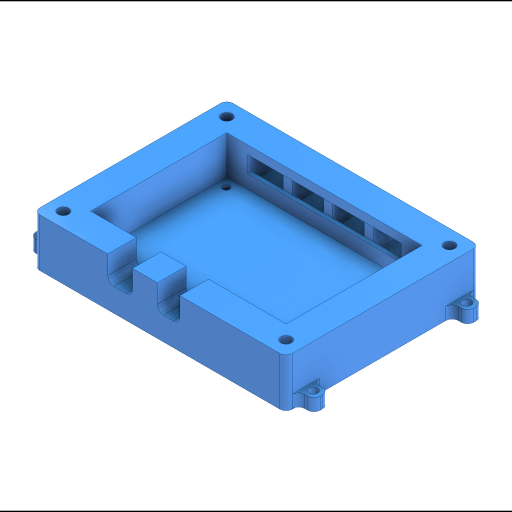
# Autodesk Inventor part: PowerBoardCase
Saved by Autodesk Inventor 2023 (Build 270158000, 158)
## iProperties
Created: 2022-02-06
Part Number: PowerBoardCase
Material: Generic
Document SubType Name: Modeling
Designer: kamer
Density: 1 g/cm^3
Appearance: Cyan
Author: kamer
## iProperties of the stored document _3DPrint.ipt
Created: 2022-02-06
Part Number: _3DPrint
Material: Generic
Document SubType Name: Modeling
Designer: kamer
Density: 1 g/cm^3
Appearance: Default
Author: kamer
Autodesk Inventor part; units mm, degrees
ref_plane "YZ Plane" through (0, 0, 0) normal (1, 0, 0) x (0, 1, 0)
ref_plane "XZ Plane" through (0, 0, 0) normal (0, 1, 0) x (-1, 0, 0)
ref_plane "XY Plane" through (0, 0, 0) normal (0, 0, 1) x (1, 0, 0)
sketch "Sketch1" plane through (0, 0, 0) normal (0, 1, 0) x (-1, 0, 0)
  line L0 (0, 0) -> (-100.33, 0)
  line L1 (-100.33, 0) -> (-100.33, -69.85)
  line L2 (-100.33, -69.85) -> (0, -69.85)
  line L3 (0, -69.85) -> (0, 0)
  line L4 (2, -71.85) -> (-102.33, -71.85)
  line L5 (-102.33, -71.85) -> (-102.33, 2)
  line L6 (-102.33, 2) -> (2, 2)
  line L7 (2, 2) -> (2, -71.85)
  dimension "d0" = 100.33
  dimension "d1" = 69.85
  dimension "d3" = 2
  dimension "d4" = 2
  dimension "d5" = 2
  dimension "d6" = 2
  constraints: 16 end point, 4 parallel, 2 horizontal, 2 perpendicular
  measures "d0" distance of L2.end L1.end
  measures "d1" distance of L1.end L0.end
  measures "d3" distance between parallel lines of L2 L4
  measures "d4" distance between parallel lines of L1 L5
  measures "d5" distance between parallel lines of L7 L3
  measures "d6" distance between parallel lines of L0 L6
extrude "Extrusion1" add sketch "Sketch1" along normal blind 7.112
sketch "Sketch2" plane through (0, 0, 0) normal (0, -1, 0) x (1, 0, 0)
  line L0 (-2, 2) -> (102.33, 2) projected
  line L1 (-2, -71.85) -> (-2, 2) projected
  line L2 (102.33, -71.85) -> (-2, -71.85) projected
  line L3 (102.33, 2) -> (102.33, -71.85) projected
  line L4 (100.33, 0) -> (0, 0) projected
  line L5 (100.33, -69.85) -> (100.33, 0) projected
  line L6 (0, -69.85) -> (100.33, -69.85) projected
  line L7 (0, 0) -> (0, -69.85) projected
extrude "Extrusion2" add sketch "Sketch2" along normal blind 5 contours L0 L3 L2 L1 | L5 L6 L7 L4
sketch "Sketch3" plane through (0, -5, 0) normal (0, -1, 0) x (1, 0, 0)
  circle A0 centre (96.4565, -65.183) radius 3.81
  circle A1 centre (4.3815, -65.183) radius 3.81
  circle A2 centre (4.3754, -4.858) radius 3.81
  circle A3 centre (96.4504, -4.858) radius 3.81
  line L0 (-2, 2) -> (-2, -71.85) projected
  line L1 (102.33, 2) -> (-2, 2) projected
  point P0 (0, 0)
  dimension "d11" = 7.62
  dimension "d12" = 7.62
  dimension "d13" = 7.62
  dimension "d14" = 7.62
  dimension "d15" = 60.325
  dimension "d16" = 60.325
  dimension "d17" = 0
  dimension "d18" = 92.075
  dimension "d19" = 92.075
  dimension "d20" = 6.3815
  dimension "d21" = 6.3754
  dimension "d22" = 6.858
  constraints: 4 centre point
  measures "d11" diameter of A0
  measures "d12" diameter of A1
  measures "d13" diameter of A2
  measures "d14" diameter of A3
  measures "d15" distance of A3.centre A0.centre
  measures "d16" distance of A2.centre A1.centre
  measures "d17" vertical distance of A1.centre A0.centre
  measures "d18" distance of A1.centre A0.centre
  measures "d19" distance of A2.centre A3.centre
  measures "d20" distance from line of A1.centre L0
  measures "d21" distance from line of L0 A2.centre
  measures "d22" distance from line of L1 A2.centre
extrude "Extrusion3" cut sketch "Sketch3" against normal blind 3.8
sketch "Sketch4" plane through (96.4565, -1.2, -65.183) normal (0, -1, 0) x (1, 0, 0)
  circle A0 centre (0, 0) radius 3.81 projected
  circle A1 centre (-0.0061, 60.325) radius 3.81 projected
  circle A2 centre (-92.0811, 60.325) radius 3.81 projected
  circle A3 centre (-92.075, 0) radius 3.81 projected
  circle A4 centre (0, 0) radius 1.778
  circle A5 centre (-92.075, 0) radius 1.778
  circle A6 centre (-92.0811, 60.325) radius 1.778
  circle A7 centre (-0.0061, 60.325) radius 1.778
  point P0 (-96.4565, 65.183)
  dimension "d25" = 3.556
  dimension "d26" = 3.556
  dimension "d27" = 3.556
  dimension "d28" = 3.556
  constraints: 4 centre point, 4 coincident
  measures "d25" diameter of A4
  measures "d26" diameter of A5
  measures "d27" diameter of A6
  measures "d28" diameter of A7
extrude "Extrusion4" cut sketch "Sketch4" against normal through all contours A4 | A5 | A6 | A7
sketch "Sketch5" plane through (0, 0, 0) normal (0, 1, 0) x (1, 0, 0)
  line L0 (9.525, 60.325) -> (90.805, 60.325)
  line L1 (90.805, 60.325) -> (90.805, 9.525)
  line L2 (90.805, 9.525) -> (9.525, 9.525)
  line L3 (9.525, 9.525) -> (9.525, 60.325)
  line L4 (0, 0) -> (0, 69.85) projected
  line L5 (0, 69.85) -> (100.33, 69.85) projected
  line L6 (100.33, 69.85) -> (100.33, 0) projected
  line L7 (100.33, 0) -> (0, 0) projected
  dimension "d31" = 9.525
  dimension "d32" = 9.525
  dimension "d33" = 9.525
  dimension "d34" = 9.525
  constraints: 8 end point, 2 parallel, 1 horizontal, 1 perpendicular
  measures "d31" distance between parallel lines of L4 L3
  measures "d32" distance between parallel lines of L5 L0
  measures "d33" distance between parallel lines of L6 L1
  measures "d34" distance between parallel lines of L7 L2
extrude "Extrusion5" cut sketch "Sketch5" against normal through all contours L0 L1 L2 L3
sketch "Sketch6" plane through (0, 7.112, 0) normal (0, 1, 0) x (1, 0, 0)
  line L0 (-2, -2) -> (102.33, -2) projected
  line L1 (102.33, -2) -> (102.33, 71.85) projected
  line L2 (102.33, 71.85) -> (-2, 71.85) projected
  line L3 (-2, 71.85) -> (-2, -2) projected
  line L4 (100.33, 0) -> (0, 0) projected
  line L5 (0, 0) -> (0, 69.85) projected
  line L6 (0, 69.85) -> (100.33, 69.85) projected
  line L7 (100.33, 69.85) -> (100.33, 0) projected
  line L8 (-2, 71.85) -> (102.33, 71.85) projected
  line L9 (0, 69.85) -> (100.33, 69.85) projected
  line L10 (10.7, 71.85) -> (89.63, 71.85)
  line L11 (89.63, 71.85) -> (89.63, 69.85)
  line L12 (89.63, 69.85) -> (10.7, 69.85)
  line L13 (10.7, 69.85) -> (10.7, 71.85)
  line L14 (100.33, 0) -> (0, 0) projected
  line L15 (23.4, 0) -> (36.1, 0)
  line L16 (36.1, 0) -> (36.1, -2)
  line L17 (36.1, -2) -> (23.4, -2)
  line L18 (23.4, -2) -> (23.4, 0)
  line L19 (48.99, 0) -> (60.42, 0)
  line L20 (60.42, 0) -> (60.42, -2)
  line L21 (60.42, -2) -> (48.99, -2)
  line L22 (48.99, -2) -> (48.99, 0)
  point P0 (10.7, 69.85)
  dimension "d37" = 12.7
  dimension "d38" = 12.7
  dimension "d39" = 12.7
  dimension "d40" = 25.4
  dimension "d41" = 41.91
  dimension "d42" = 11.43
  constraints: 24 end point, 6 parallel, 6 point on line, 3 horizontal, 3 perpendicular
  measures "d37" distance between parallel lines of L3 L13
  measures "d38" distance between parallel lines of L1 L11
  measures "d39" distance between parallel lines of L16 L18
  measures "d40" distance between parallel lines of L3 L18
  measures "d41" distance between parallel lines of L1 L20
  measures "d42" distance between parallel lines of L22 L20
extrude "Extrusion6" add sketch "Sketch6" along normal blind 12.7 contours L3 L2 L13 L6 L5 L4 L18 L0 | L16 L4 L22 L0 | L2 L1 L0 L20 L4 L7 L6 L11
sketch "Sketch7" plane through (9.525, 0, -9.525) normal (1, 0, 0) x (0, 0, -1)
  line L0 (50.8, -5) -> (0, -5) projected
  line L1 (50.8, 0) -> (50.8, -5) projected
  line L2 (0, 0) -> (50.8, 0) projected
  line L3 (0, 0) -> (0, -5) projected
  point P0 (-9.525, 0)
extrude "Extrusion7" add sketch "Sketch7" along normal up to surface (81.28 mm away)
sketch "Sketch12" plane through (102.33, -5, 2) normal (1, 0, 0) x (0, 0, -1)
  line L0 (0, 0) -> (0, 24.812) projected
  line L1 (73.85, 0) -> (73.85, 24.812) projected
  line L2 (0, 24.812) -> (73.85, 24.812)
  line L3 (73.85, 24.812) -> (73.85, 0)
  line L4 (73.85, 0) -> (0, 0)
  line L5 (0, 0) -> (0, 24.812)
  point P0 (2, 5)
  constraints: 8 end point, 2 parallel, 1 horizontal, 1 perpendicular
extrude "Extrusion12" add sketch "Sketch12" along normal blind 12.7
sketch "Sketch13" plane through (-2, -5, -71.85) normal (-1, 0, 0) x (0, 0, 1)
  line L0 (73.85, 24.812) -> (73.85, 0) projected
  line L1 (0, 24.812) -> (73.85, 24.812) projected
  line L2 (0, 0) -> (0, 24.812) projected
  line L3 (73.85, 0) -> (0, 0) projected
  point P0 (71.85, 5)
extrude "Extrusion13" add sketch "Sketch13" along normal blind 12.7
sketch "Sketch14" plane through (36.1, 19.812, 2) normal (0, 0, 1) x (1, 0, 0)
  line L0 (24.32, 0) -> (78.93, 0) projected
  line L1 (24.32, -12.7) -> (24.32, 0) projected
  line L2 (12.89, -12.7) -> (24.32, -12.7) projected
  line L3 (12.89, -12.7) -> (12.89, 0) projected
  line L4 (0, 0) -> (12.89, 0) projected
  line L5 (0, -12.7) -> (0, 0) projected
  line L6 (-12.7, -12.7) -> (0, -12.7) projected
  line L7 (-12.7, -12.7) -> (-12.7, 0) projected
  line L8 (-12.7, 0) -> (-50.8, 0) projected
  line L9 (-50.8, -24.812) -> (-50.8, 0) projected
  line L10 (-50.8, -24.812) -> (78.93, -24.812) projected
  line L11 (78.93, 0) -> (78.93, -24.812) projected
  point P0 (-36.1, -19.812)
extrude "Extrusion14" add sketch "Sketch14" along normal blind 12.7
sketch "Sketch16" plane through (89.63, 7.112, -71.85) normal (0, 0, -1) x (-1, 0, 0)
  line L0 (78.93, 12.7) -> (104.33, 12.7) projected
  line L1 (78.93, 0) -> (78.93, 12.7) projected
  line L2 (0, 0) -> (78.93, 0) projected
  line L3 (0, 0) -> (0, 12.7) projected
  line L4 (0, 12.7) -> (-25.4, 12.7) projected
  line L5 (-25.4, -12.112) -> (-25.4, 12.7) projected
  line L6 (-25.4, -12.112) -> (104.33, -12.112) projected
  line L7 (104.33, 12.7) -> (104.33, -12.112) projected
  line L8 (78.93, 0) -> (0, 0) projected
  line L9 (0, 0) -> (78.93, 0)
  line L10 (78.93, 0) -> (78.93, -4.492)
  line L11 (78.93, -4.492) -> (0, -4.492)
  line L12 (0, -4.492) -> (0, 0)
  point P0 (89.63, -7.112)
  dimension "d86" = 7.62
  constraints: 8 end point, 2 parallel, 1 horizontal, 1 perpendicular
  measures "d86" distance between parallel lines of L6 L11
extrude "Extrusion16" add sketch "Sketch16" along normal blind 12.7 contours L0 L7 L6 L5 L4 L3 L12 L11 L10 L1
sketch "Sketch17" plane through (0, 19.812, 0) normal (0, 1, 0) x (1, 0, 0)
  point P0 (0, 0)
sketch "Sketch18" plane through (89.63, 7.112, -71.85) normal (-1, 0, 0) x (0, 0, 1)
  line L0 (-12.7, -4.492) -> (-12.7, 12.7) projected
  line L1 (2, 0) -> (2, 12.7) projected
  line L2 (-12.7, 12.7) -> (2, 12.7)
  line L3 (2, 12.7) -> (2, 8.382)
  line L4 (2, 8.382) -> (-12.7, 8.382)
  line L5 (-12.7, 8.382) -> (-12.7, 12.7)
  point P0 (71.85, -7.112)
  point P1 (-12.7, 8.382)
  dimension "d89" = 4.318
  constraints: 8 end point, 2 parallel, 1 horizontal, 1 perpendicular, 1 point on line
  measures "d89" distance between parallel lines of L2 L4
extrude "Extrusion17" add sketch "Sketch18" along normal up to surface (78.93 mm away)
sketch "Sketch19" plane through (89.63, 7.112, -71.85) normal (0, 0, -1) x (-1, 0, 0)
  line L0 (0, 0) -> (78.93, 0) projected
  line L1 (0, 8.382) -> (78.93, 8.382) projected
  line L2 (39.465, 0) -> (41.8145, 0)
  line L3 (41.8145, 0) -> (41.8145, 8.382)
  line L4 (41.8145, 8.382) -> (39.465, 8.382)
  line L5 (39.465, 8.382) -> (39.465, 0)
  line L6 (39.465, 0) -> (37.1155, 0)
  line L7 (37.1155, 0) -> (37.1155, 8.382)
  line L8 (37.1155, 8.382) -> (39.465, 8.382)
  line L9 (39.465, 8.382) -> (39.465, 0)
  line L10 (78.93, 0) -> (0, 0) projected
  line L11 (57.9435, 0) -> (62.6425, 0)
  line L12 (62.6425, 0) -> (62.6425, 8.382)
  line L13 (62.6425, 8.382) -> (57.9435, 8.382)
  line L14 (57.9435, 8.382) -> (57.9435, 0)
  line L15 (20.9865, 0) -> (16.2875, 0)
  line L16 (16.2875, 0) -> (16.2875, 8.382)
  line L17 (16.2875, 8.382) -> (20.9865, 8.382)
  line L18 (20.9865, 8.382) -> (20.9865, 0)
  line L19 (0, -4.492) -> (78.93, -4.492) projected
  line L20 (16.2875, 0) -> (20.9865, 0)
  line L21 (20.9865, 0) -> (20.9865, -4.492)
  line L22 (20.9865, -4.492) -> (16.2875, -4.492)
  line L23 (16.2875, -4.492) -> (16.2875, 0)
  line L24 (37.1155, 0) -> (41.8145, 0)
  line L25 (41.8145, 0) -> (41.8145, -4.492)
  line L26 (41.8145, -4.492) -> (37.1155, -4.492)
  line L27 (37.1155, -4.492) -> (37.1155, 0)
  line L28 (57.9435, 0) -> (62.6425, 0)
  line L29 (62.6425, 0) -> (62.6425, -4.492)
  line L30 (62.6425, -4.492) -> (57.9435, -4.492)
  line L31 (57.9435, -4.492) -> (57.9435, 0)
  point P0 (89.63, -7.112)
  point P1 (37.1155, 4.191)
  point P2 (62.6425, -4.492)
  point P3 (62.6425, 0)
  point P4 (37.1155, -4.492)
  point P5 (41.8145, -4.492)
  point P6 (41.8145, 0)
  point P7 (37.1155, 8.382)
  point P8 (16.2875, -4.492)
  point P9 (20.9865, 0)
  point P10 (20.9865, 8.382)
  dimension "d92" = 2.3495
  dimension "d93" = 2.3495
  dimension "d94" = 16.129
  dimension "d95" = 4.699
  dimension "d96" = 4.699
  dimension "d97" = 16.129
  constraints: 56 end point, 14 parallel, 9 point on line, 7 horizontal, 7 perpendicular, 2 midpoint
  measures "d92" distance between parallel lines of L7 L5
  measures "d93" distance between parallel lines of L5 L3
  measures "d94" distance between parallel lines of L14 L3
  measures "d95" distance between parallel lines of L14 L12
  measures "d96" distance between parallel lines of L16 L18
  measures "d97" distance from line of point (37.116, 4.191) L18
extrude "Extrusion18" add sketch "Sketch19" along normal up to surface (12.7 mm away) contours L16 L1 L18 L0 | L0 L21 L19 L23 | L7 L1 L5 L0 | L0 L25 L19 L27 | L5 L1 L3 L0 | L14 L1 L12 L0 | L0 L29 L19 L31
fillet "Fillet3" radius 3.175 4 edges at (23.4, 7.112, 7.35) (36.1, 7.112, 7.35) (48.99, 7.112, 7.35) (60.42, 7.112, 7.35)
fillet "Fillet4" radius 3.175 4 edges at (-14.7, 7.406, 14.7) (-14.7, 7.406, -84.55) (115.03, 7.406, -84.55) (115.03, 7.406, 14.7)
sketch "Sketch20" plane through (0, 19.812, 0) normal (0, 1, 0) x (1, 0, 0)
  circle A0 centre (-7.08, 76.93) radius 2.7559
  circle A1 centre (107.41, 76.93) radius 2.7559
  circle A2 centre (107.41, -7.08) radius 2.7559
  circle A3 centre (-7.08, -7.08) radius 2.7559
  line L0 (-14.7, 81.375) -> (-14.7, -11.525) projected
  line L1 (115.03, -11.525) -> (115.03, 81.375) projected
  line L2 (23.4, -14.7) -> (-11.525, -14.7) projected
  line L3 (-11.525, 84.55) -> (111.855, 84.55) projected
  line L4 (111.855, -14.7) -> (60.42, -14.7) projected
  point P0 (0, 0)
  dimension "d102" = 5.5118
  dimension "d103" = 5.5118
  dimension "d104" = 5.5118
  dimension "d105" = 5.5118
  dimension "d106" = 7.62
  dimension "d107" = 7.62
  dimension "d108" = 7.62
  dimension "d109" = 7.62
  dimension "d110" = 7.62
  dimension "d111" = 7.62
  dimension "d112" = 7.62
  dimension "d113" = 7.62
  constraints: 4 centre point
  measures "d102" diameter of A0
  measures "d103" diameter of A1
  measures "d104" diameter of A2
  measures "d105" diameter of A3
  measures "d106" distance from line of L0 A3.centre
  measures "d107" distance from line of L0 A0.centre
  measures "d108" distance from line of L1 A1.centre
  measures "d109" distance from line of L2 A3.centre
  measures "d110" distance from line of L3 A0.centre
  measures "d111" distance from line of L3 A1.centre
  measures "d112" distance from line of L1 A2.centre
  measures "d113" distance from line of L4 A2.centre
extrude "Extrusion19" cut sketch "Sketch20" against normal blind 12.7
sketch "Sketch21" plane through (115.03, -5, 2) normal (1, 0, 0) x (0, 0, -1)
  line L0 (-6.35, 6.6675) -> (1.27, 6.6675)
  line L1 (1.27, 6.6675) -> (1.27, 0.3175)
  line L2 (1.27, 0.3175) -> (-6.35, 0.3175)
  line L3 (-6.35, 0.3175) -> (-6.35, 6.6675)
  line L4 (83.375, 0) -> (-9.525, 0) projected
  line L5 (80.2, 0) -> (72.58, 0)
  line L6 (72.58, 0) -> (72.58, 6.35)
  line L7 (72.58, 6.35) -> (80.2, 6.35)
  line L8 (80.2, 6.35) -> (80.2, 0)
  line L9 (-12.7, 24.812) -> (-12.7, 0) projected
  line L10 (86.55, 0) -> (86.55, 24.812) projected
  point P0 (2, 5)
  dimension "d116" = 7.62
  dimension "d117" = 6.35
  dimension "d118" = 7.62
  dimension "d119" = 6.35
  dimension "d120" = 6.35
  dimension "d121" = 6.35
  constraints: 16 end point, 4 parallel, 2 horizontal, 2 perpendicular, 1 point on line
  measures "d116" distance of L1.end L2.end
  measures "d117" distance of L0.end L1.end
  measures "d118" distance of L6.end L7.end
  measures "d119" distance of L5.end L6.end
  measures "d120" distance between parallel lines of L3 L9
  measures "d121" distance between parallel lines of L10 L8
extrude "Extrusion20" add sketch "Sketch21" along normal blind 7.9375 and the other way blind 138.1252
sketch "Sketch22" plane through (-23.0952, 1.35, -78.2) normal (0, 1, 0) x (1, 0, 0)
  circle A0 centre (4.5852, -3.81) radius 2.286
  circle A1 centre (141.9352, -3.81) radius 2.286
  circle A2 centre (141.9352, -82.74) radius 2.286
  circle A3 centre (4.5852, -82.74) radius 2.286
  line L0 (8.3952, 3.175) -> (8.3952, -89.725) projected
  line L1 (0, 0) -> (8.3952, 0) projected
  line L2 (0, -86.55) -> (8.3952, -86.55) projected
  line L3 (138.1252, -89.725) -> (138.1252, 3.175) projected
  line L4 (138.1252, -78.93) -> (146.0627, -78.93) projected
  line L5 (146.0627, -7.62) -> (138.1252, -7.62) projected
  point P0 (23.0952, -78.2)
  point P1 (142.0939, -78.93)
  dimension "d126" = 3.81
  dimension "d127" = 3.81
  dimension "d128" = 3.81
  dimension "d129" = 3.81
  dimension "d130" = 4.572
  dimension "d131" = 4.572
  dimension "d132" = 4.572
  dimension "d133" = 3.81
  dimension "d134" = 3.81
  dimension "d135" = 4.572
  dimension "d136" = 3.81
  dimension "d137" = 3.81
  constraints: 4 centre point, 1 midpoint
  measures "d126" distance from line of L0 A3.centre
  measures "d127" distance from line of L0 A0.centre
  measures "d128" distance from line of L1 A0.centre
  measures "d129" distance from line of L2 A3.centre
  measures "d130" diameter of A0
  measures "d131" diameter of A3
  measures "d132" diameter of A2
  measures "d133" distance from line of L3 A2.centre
  measures "d134" vertical distance of point (142.094, -78.93) A2.centre
  measures "d135" diameter of A1
  measures "d136" distance from line of L5 A1.centre
  measures "d137" distance from line of L3 A1.centre
extrude "Extrusion21" cut sketch "Sketch22" along normal through all both and the other way through all
fillet "Fillet5" radius 3.175 16 edges at (115.03, -1.825, -70.58) (122.9675, -1.825, -70.58) (122.9675, -1.825, -78.2) (115.03, -1.5075, 8.35) (122.9675, -1.5075, 8.35) (122.9675, -1.5075, 0.73) (115.03, -1.5075, 0.73) (115.03, -1.825, -78.2) (-14.7, -1.5075, 8.35) (-14.7, -1.5075, 0.73) (-23.0952, -1.5075, 8.35) (-23.0952, -1.5075, 0.73) (-14.7, -1.825, -78.2) (-14.7, -1.825, -70.58) (-23.0952, -1.825, -70.58) (-23.0952, -1.825, -78.2)
body "Solid1"
